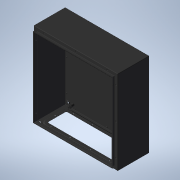
# Autodesk Inventor part: 1050.000(1)_P1
Saved by Autodesk Inventor 2021 (Build 250183000, 183)
## iProperties
Created: 2025-07-29
Part Number: 1050.000(1)_P1
Material: Generic
Catalog Web Link: www.cadenas.de
Description: AE 2.0 Gehaeuse-AE 2.0 Gehaeuse
Vendor: RITTAL
Document SubType Name: Modeling
Designer: psAdmin
Manufacturer: RITTAL
Mass: 833.937 g
Surface Area: 13154.2 cm^2
Volume: 833.937 cm^3
Density: 1 g/cm^3
Appearance: PSOLRGB-176-176-176
Category: PARTsolutions
Company: RITTAL
Title: 1050.000(1)_P1
Author: Cadenas PARTsolutions
Comments: AE 2.0 Gehaeuse
PSOL_IDENT_0: {$CADENAS_DATA/23d-libs/rittal/schaltschranksys/kompakt_schaltschr/parts_ae_2_0/gehaeuse_ae_2_0.prj}
PSOL_IDENT_1: ,190 {VTYP=3D},{NB=1050.000(1)_P1},{LINA=1050.000(1)_P1},{NN=AE 2.0 Gehaeuse},{DATE=25.07.2025 12:41
PSOL_IDENT_2: :23},{GEOMDATE=24.07.2025 05:50:00},{VERSION=},{LINEID=180},{WBVAR=DETAIL},{WBNUMERIC=DETAIL}  {NB=1
PSOL_IDENT_3: 050.000(1)_P1},{LINA=1050.000(1)_P1},{KT=DUMMY},{DETAIL=1},{BEZ1=Neues Kompaktgehäuse},{BEZ2=Stahlbl
PSOL_IDENT_4: ech},{BEZ3=eintürig},{TUER=1},{B=500},{H=500},{T=210},{F=450},{G=475},{B1=500},{BEST=1050.000},{B3=4
PSOL_IDENT_5: 60.000},{B4=383.000},{B5=411.000},{BB5=0.000},{H1=500},{H3=460.000},{H4=85.000},{H5=113.000},{HH5=4.
PSOL_IDENT_6: 000},{T5=93.500},{R1=31.000},{R2=8.000},{T1=210},{F1=450},{G1=475},{VERS3=0},{VERS=4},{CNSECLASS51=2
PSOL_IDENT_7: 7-18-01-02},{CNSECLASS70=27-18-01-01},{CNSECLASS80=27-18-01-01},{CNSETIM40=EC000261},{S=1.25},{W=500
PSOL_IDENT_8: .000},{W1=456.500},{W2=400.000},{HH=500.000},{HH1=456.500},{HH2=450.000},{HH3=375.000},{D=187.000},{
PSOL_IDENT_9: D1=204.300},{VERS1=1},{GEW=15,42},{CNSETIM80=EC000261},{CNSETIM90=EC000261},{CNSECLASS60=27-18-01-01
PSOL_IDENT_10: },{UNSPSC=31-26-15-02}
NB: 1050.000(1)_P1
NN: AE 2.0 Gehaeuse
NT: AE 2.0 Gehaeuse
NBSYN: $BEST.($DETAIL.)_P1
LINA: 1050.000(1)_P1
CATALOG: Rittal
DETAIL: hoch
BEZ1: Neues Kompaktgehäuse
BEZ2: Stahlblech
BEZ3: eintürig
TUER: 1
B: 500
H: 500
T: 210
F: 450
G: 475
B1: 500
BEST: 1050.000
B3: 460
B4: 383
B5: 411
BB5: 0
H1: 500
H3: 460
H4: 85
H5: 113
HH5: 4
T5: 93.5
R1: 31
R2: 8
T1: 210
F1: 450
G1: 475
VERS3: 0
VERS: 4
CNSECLASS70: 27-18-01-01
CNSECLASS80: 27-18-01-01
S: 1.25
W: 500
W1: 456.5
W2: 400
HH: 500
HH1: 456.5
HH2: 450
HH3: 375
D: 187
D1: 204.3
VERS1: 1
GEW: 15,42
CNSETIM80: EC000261
CNSETIM90: EC000261
CNSECLASS60: 27-18-01-01
UNSPSC: 31-26-15-02
SUPPLIER: RITTAL
ARTICLENO: 1050.000(1)_P1
BOMINFO: 1050.000(1)_P1
CREATOR: CADENAS GmbH
Autodesk Inventor part; units mm, degrees
(part 1 of 2)
sketch "Sketch_1" plane through (0, 0, 0) normal (0, 1, 0) x (1, 0, 0)
  line L0 (-250, -82) -> (250, -82)
  line L1 (250, -82) -> (250, 105)
  line L2 (250, 105) -> (-250, 105)
  line L3 (-250, 105) -> (-250, -82)
  arc A0 (-248.75, -79.5) -> (-247.5, -80.75) centre (-247.5, -79.5) ccw
  line L4 (-247.5, -80.75) -> (247.5, -80.75)
  arc A1 (247.5, -80.75) -> (248.75, -79.5) centre (247.5, -79.5) ccw
  line L5 (248.75, -79.5) -> (248.75, 102.5)
  arc A2 (248.75, 102.5) -> (247.5, 103.75) centre (247.5, 102.5) ccw
  line L6 (247.5, 103.75) -> (-247.5, 103.75)
  arc A3 (-247.5, 103.75) -> (-248.75, 102.5) centre (-247.5, 102.5) ccw
  line L7 (-248.75, 102.5) -> (-248.75, -79.5)
  constraints: 16 end point, 8 point on circle, 4 centre point
extrude "Extrusion1" add sketch "Sketch_1" along normal blind 500
sketch "Sketch_2" plane through (0, 0, 82) normal (0, 0, 1) x (1, 0, 0)
  line L0 (-230.75, 19.25) -> (230.75, 19.25)
  line L1 (230.75, 19.25) -> (230.75, 480.75)
  line L2 (230.75, 480.75) -> (-230.75, 480.75)
  line L3 (-230.75, 480.75) -> (-230.75, 19.25)
  constraints: 8 end point
extrude "Extrusion2" cut sketch "Sketch_2" against normal blind 1.25
sketch "Sketch_3" plane through (0, 0, 0) normal (1, 0, 0) x (0, 0, -1)
  line L0 (-82, 490) -> (-80.75, 490)
  line L1 (-80.75, 490) -> (-80.75, 497.5)
  arc A0 (-79.5, 498.75) -> (-80.75, 497.5) centre (-79.5, 497.5) ccw
  line L2 (-79.5, 498.75) -> (102.5, 498.75)
  arc A1 (103.75, 497.5) -> (102.5, 498.75) centre (102.5, 497.5) ccw
  line L3 (103.75, 497.5) -> (103.75, 2.5)
  arc A2 (102.5, 1.25) -> (103.75, 2.5) centre (102.5, 2.5) ccw
  line L4 (102.5, 1.25) -> (-79.5, 1.25)
  arc A3 (-80.75, 2.5) -> (-79.5, 1.25) centre (-79.5, 2.5) ccw
  line L5 (-80.75, 2.5) -> (-80.75, 10)
  line L6 (-80.75, 10) -> (-82, 10)
  line L7 (-82, 10) -> (-82, 0)
  line L8 (-82, 0) -> (105, 0)
  line L9 (105, 0) -> (105, 500)
  line L10 (105, 500) -> (-82, 500)
  line L11 (-82, 500) -> (-82, 490)
  constraints: 24 end point, 8 point on circle, 4 centre point
extrude "Extrusion3" add sketch "Sketch_3" along normal mid plane 500
sketch "Sketch_4" plane through (0, 0, 0) normal (1, 0, 0) x (0, 0, -1)
  line L0 (-83.25, 501.25) -> (-83.25, -1.25)
  line L1 (-83.25, -1.25) -> (106.25, -1.25)
  line L2 (106.25, -1.25) -> (106.25, 501.25)
  line L3 (106.25, 501.25) -> (-83.25, 501.25)
  line L4 (-82, 497.5) -> (-82, 2.5)
  arc A0 (-82, 2.5) -> (-79.5, 0) centre (-79.5, 2.5) ccw
  line L5 (-79.5, 0) -> (102.5, 0)
  arc A1 (102.5, 0) -> (105, 2.5) centre (102.5, 2.5) ccw
  line L6 (105, 2.5) -> (105, 497.5)
  arc A2 (105, 497.5) -> (102.5, 500) centre (102.5, 497.5) ccw
  line L7 (102.5, 500) -> (-79.5, 500)
  arc A3 (-79.5, 500) -> (-82, 497.5) centre (-79.5, 497.5) ccw
  constraints: 16 end point, 8 point on circle, 4 centre point
extrude "Extrusion4" cut sketch "Sketch_4" along normal mid plane 500
sketch "Sketch_5" plane through (0, 0, 0) normal (0, 1, 0) x (1, 0, 0)
  line L0 (-251.25, -83.25) -> (251.25, -83.25)
  line L1 (251.25, -83.25) -> (251.25, 106.25)
  line L2 (251.25, 106.25) -> (-251.25, 106.25)
  line L3 (-251.25, 106.25) -> (-251.25, -83.25)
  arc A0 (-250, -79.5) -> (-247.5, -82) centre (-247.5, -79.5) ccw
  line L4 (-247.5, -82) -> (247.5, -82)
  arc A1 (247.5, -82) -> (250, -79.5) centre (247.5, -79.5) ccw
  line L5 (250, -79.5) -> (250, 102.5)
  arc A2 (250, 102.5) -> (247.5, 105) centre (247.5, 102.5) ccw
  line L6 (247.5, 105) -> (-247.5, 105)
  arc A3 (-247.5, 105) -> (-250, 102.5) centre (-247.5, 102.5) ccw
  line L7 (-250, 102.5) -> (-250, -79.5)
  constraints: 16 end point, 8 point on circle, 4 centre point
extrude "Extrusion5" cut sketch "Sketch_5" along normal blind 500
sketch "Sketch_48" plane through (0, 0, -105) normal (0, 0, 1) x (1, 0, 0)
  line L0 (-246.25, 496.25) -> (-246.25, 3.75)
  line L1 (-246.25, 3.75) -> (246.25, 3.75)
  line L2 (246.25, 3.75) -> (246.25, 496.25)
  line L3 (246.25, 496.25) -> (-246.25, 496.25)
  constraints: 8 end point
extrude "Extrusion6" cut sketch "Sketch_48" along normal blind 1.25
sketch "Sketch_49" plane through (0, 0, -105) normal (0, 0, 1) x (1, 0, 0)
  line L0 (-246.25, 496.25) -> (-246.25, 3.75)
  line L1 (-246.25, 3.75) -> (246.25, 3.75)
  line L2 (246.25, 3.75) -> (246.25, 496.25)
  line L3 (246.25, 496.25) -> (-246.25, 496.25)
  line L4 (218.5, 8.5) -> (241.5, 8.5)
  line L5 (241.5, 8.5) -> (241.5, 31.5)
  line L6 (241.5, 31.5) -> (218.5, 31.5)
  line L7 (218.5, 31.5) -> (218.5, 8.5)
  line L8 (218.5, 468.5) -> (241.5, 468.5)
  line L9 (241.5, 468.5) -> (241.5, 491.5)
  line L10 (241.5, 491.5) -> (218.5, 491.5)
  line L11 (218.5, 491.5) -> (218.5, 468.5)
  line L12 (-241.5, 8.5) -> (-218.5, 8.5)
  line L13 (-218.5, 8.5) -> (-218.5, 31.5)
  line L14 (-218.5, 31.5) -> (-241.5, 31.5)
  line L15 (-241.5, 31.5) -> (-241.5, 8.5)
  line L16 (-241.5, 468.5) -> (-218.5, 468.5)
  line L17 (-218.5, 468.5) -> (-218.5, 491.5)
  line L18 (-218.5, 491.5) -> (-241.5, 491.5)
  line L19 (-241.5, 491.5) -> (-241.5, 468.5)
  constraints: 40 end point
extrude "Extrusion7" add sketch "Sketch_49" along normal blind 1.25
sketch "Sketch_105" plane through (0, 0, -105) normal (0, 0, 1) x (1, 0, 0)
  line L0 (-270, 520) -> (-270, -20)
  line L1 (-270, -20) -> (270, -20)
  line L2 (270, -20) -> (270, 520)
  line L3 (270, 520) -> (-270, 520)
  line L4 (-250, 497.5) -> (-250, 2.5)
  arc A0 (-250, 2.5) -> (-247.5, 0) centre (-247.5, 2.5) ccw
  line L5 (-247.5, 0) -> (247.5, 0)
  arc A1 (247.5, 0) -> (250, 2.5) centre (247.5, 2.5) ccw
  line L6 (250, 2.5) -> (250, 497.5)
  arc A2 (250, 497.5) -> (247.5, 500) centre (247.5, 497.5) ccw
  line L7 (247.5, 500) -> (-247.5, 500)
  arc A3 (-247.5, 500) -> (-250, 497.5) centre (-247.5, 497.5) ccw
  constraints: 16 end point, 8 point on circle, 4 centre point
extrude "Extrusion8" cut sketch "Sketch_105" along normal blind 210
sketch "Sketch_50" plane through (0, 20, 0) normal (0, 1, 0) x (1, 0, 0)
  line L0 (-241.5, 103.75) -> (-240.1443, 103.75)
  line L1 (-240.1443, 103.75) -> (-238.9896, 101.75)
  line L2 (-238.9896, 101.75) -> (-221.0104, 101.75)
  line L3 (-221.0104, 101.75) -> (-219.8557, 103.75)
  line L4 (-219.8557, 103.75) -> (-218.5, 103.75)
  line L5 (-218.5, 103.75) -> (-218.5, 105)
  line L6 (-218.5, 105) -> (-220, 105)
  line L7 (-220, 105) -> (-221.1547, 103)
  line L8 (-221.1547, 103) -> (-238.8453, 103)
  line L9 (-238.8453, 103) -> (-240, 105)
  line L10 (-240, 105) -> (-241.5, 105)
  line L11 (-241.5, 105) -> (-241.5, 103.75)
  constraints: 24 end point
extrude "Extrusion9" add sketch "Sketch_50" along normal mid plane 15.35
sketch "Sketch_51" plane through (0, 20, 0) normal (0, 1, 0) x (1, 0, 0)
  line L0 (218.5, 103.75) -> (219.8557, 103.75)
  line L1 (219.8557, 103.75) -> (221.0104, 101.75)
  line L2 (221.0104, 101.75) -> (238.9896, 101.75)
  line L3 (238.9896, 101.75) -> (240.1443, 103.75)
  line L4 (240.1443, 103.75) -> (241.5, 103.75)
  line L5 (241.5, 103.75) -> (241.5, 105)
  line L6 (241.5, 105) -> (240, 105)
  line L7 (240, 105) -> (238.8453, 103)
  line L8 (238.8453, 103) -> (221.1547, 103)
  line L9 (221.1547, 103) -> (220, 105)
  line L10 (220, 105) -> (218.5, 105)
  line L11 (218.5, 105) -> (218.5, 103.75)
  constraints: 24 end point
extrude "Extrusion10" add sketch "Sketch_51" along normal mid plane 15.35
sketch "Sketch_52" plane through (0, 27.675, 0) normal (0, 1, 0) x (1, 0, 0)
  line L0 (-222.325, 101.75) -> (-222.325, 103)
  line L1 (-222.325, 103) -> (-221.1547, 103)
  line L2 (-221.1547, 103) -> (-220, 105)
  line L3 (-220, 105) -> (-215.5, 105)
  line L4 (-215.5, 105) -> (-215.5, 103.75)
  line L5 (-215.5, 103.75) -> (-219.8557, 103.75)
  line L6 (-219.8557, 103.75) -> (-221.0104, 101.75)
  line L7 (-221.0104, 101.75) -> (-222.325, 101.75)
  line L8 (-222.325, 101.75) -> (-222.325, 103)
  constraints: 18 end point
revolve "Revolution1" add sketch "Sketch_52" angle 90 about axis through (-222.325, 27.675, -101.75) along (0, 0, 1)
sketch "Sketch_53" plane through (0, 27.675, 0) normal (0, 1, 0) x (1, 0, 0)
  line L0 (-237.675, 103) -> (-237.675, 101.75)
  line L1 (-237.675, 101.75) -> (-238.9896, 101.75)
  line L2 (-238.9896, 101.75) -> (-240.1443, 103.75)
  line L3 (-240.1443, 103.75) -> (-244.5, 103.75)
  line L4 (-244.5, 103.75) -> (-244.5, 105)
  line L5 (-244.5, 105) -> (-240, 105)
  line L6 (-240, 105) -> (-238.8453, 103)
  line L7 (-238.8453, 103) -> (-237.675, 103)
  line L8 (-237.675, 103) -> (-237.675, 101.75)
  constraints: 18 end point
revolve "Revolution2" add sketch "Sketch_53" angle 90 about axis through (-237.675, 27.675, -103) along (0, 0, -1)
sketch "Sketch_54" plane through (0, 27.675, 0) normal (0, 1, 0) x (1, 0, 0)
  line L0 (237.675, 101.75) -> (237.675, 103)
  line L1 (237.675, 103) -> (238.8453, 103)
  line L2 (238.8453, 103) -> (240, 105)
  line L3 (240, 105) -> (244.5, 105)
  line L4 (244.5, 105) -> (244.5, 103.75)
  line L5 (244.5, 103.75) -> (240.1443, 103.75)
  line L6 (240.1443, 103.75) -> (238.9896, 101.75)
  line L7 (238.9896, 101.75) -> (237.675, 101.75)
  line L8 (237.675, 101.75) -> (237.675, 103)
  constraints: 18 end point
revolve "Revolution3" add sketch "Sketch_54" angle 90 about axis through (237.675, 27.675, -101.75) along (0, 0, 1)
sketch "Sketch_55" plane through (0, 27.675, 0) normal (0, 1, 0) x (1, 0, 0)
  line L0 (222.325, 103) -> (222.325, 101.75)
  line L1 (222.325, 101.75) -> (221.0104, 101.75)
  line L2 (221.0104, 101.75) -> (219.8557, 103.75)
  line L3 (219.8557, 103.75) -> (215.5, 103.75)
  line L4 (215.5, 103.75) -> (215.5, 105)
  line L5 (215.5, 105) -> (220, 105)
  line L6 (220, 105) -> (221.1547, 103)
  line L7 (221.1547, 103) -> (222.325, 103)
  line L8 (222.325, 103) -> (222.325, 101.75)
  constraints: 18 end point
revolve "Revolution4" add sketch "Sketch_55" angle 90 about axis through (222.325, 27.675, -103) along (0, 0, -1)
sketch "Sketch_56" plane through (0, 12.325, 0) normal (0, 1, 0) x (1, 0, 0)
  line L0 (-222.325, 101.75) -> (-222.325, 103)
  line L1 (-222.325, 103) -> (-221.1547, 103)
  line L2 (-221.1547, 103) -> (-220, 105)
  line L3 (-220, 105) -> (-215.5, 105)
  line L4 (-215.5, 105) -> (-215.5, 103.75)
  line L5 (-215.5, 103.75) -> (-219.8557, 103.75)
  line L6 (-219.8557, 103.75) -> (-221.0104, 101.75)
  line L7 (-221.0104, 101.75) -> (-222.325, 101.75)
  line L8 (-222.325, 101.75) -> (-222.325, 103)
  constraints: 18 end point
revolve "Revolution5" add sketch "Sketch_56" angle 90 about axis through (-222.325, 12.325, -101.75) along (0, 0, -1)
sketch "Sketch_57" plane through (0, 12.325, 0) normal (0, 1, 0) x (1, 0, 0)
  line L0 (-237.675, 103) -> (-237.675, 101.75)
  line L1 (-237.675, 101.75) -> (-238.9896, 101.75)
  line L2 (-238.9896, 101.75) -> (-240.1443, 103.75)
  line L3 (-240.1443, 103.75) -> (-244.5, 103.75)
  line L4 (-244.5, 103.75) -> (-244.5, 105)
  line L5 (-244.5, 105) -> (-240, 105)
  line L6 (-240, 105) -> (-238.8453, 103)
  line L7 (-238.8453, 103) -> (-237.675, 103)
  line L8 (-237.675, 103) -> (-237.675, 101.75)
  constraints: 18 end point
revolve "Revolution6" add sketch "Sketch_57" angle 90 about axis through (-237.675, 12.325, -103) along (0, 0, 1)
sketch "Sketch_58" plane through (0, 12.325, 0) normal (0, 1, 0) x (1, 0, 0)
  line L0 (237.675, 101.75) -> (237.675, 103)
  line L1 (237.675, 103) -> (238.8453, 103)
  line L2 (238.8453, 103) -> (240, 105)
  line L3 (240, 105) -> (244.5, 105)
  line L4 (244.5, 105) -> (244.5, 103.75)
  line L5 (244.5, 103.75) -> (240.1443, 103.75)
  line L6 (240.1443, 103.75) -> (238.9896, 101.75)
  line L7 (238.9896, 101.75) -> (237.675, 101.75)
  line L8 (237.675, 101.75) -> (237.675, 103)
  constraints: 18 end point
revolve "Revolution7" add sketch "Sketch_58" angle 90 about axis through (237.675, 12.325, -101.75) along (0, 0, -1)
sketch "Sketch_59" plane through (0, 12.325, 0) normal (0, 1, 0) x (1, 0, 0)
  line L0 (222.325, 103) -> (222.325, 101.75)
  line L1 (222.325, 101.75) -> (221.0104, 101.75)
  line L2 (221.0104, 101.75) -> (219.8557, 103.75)
  line L3 (219.8557, 103.75) -> (215.5, 103.75)
  line L4 (215.5, 103.75) -> (215.5, 105)
  line L5 (215.5, 105) -> (220, 105)
  line L6 (220, 105) -> (221.1547, 103)
  line L7 (221.1547, 103) -> (222.325, 103)
  line L8 (222.325, 103) -> (222.325, 101.75)
  constraints: 18 end point
revolve "Revolution8" add sketch "Sketch_59" angle 90 about axis through (222.325, 12.325, -103) along (0, 0, 1)
sketch "Sketch_60" plane through (0, 480, 0) normal (0, 1, 0) x (1, 0, 0)
  line L0 (-241.5, 103.75) -> (-240.1443, 103.75)
  line L1 (-240.1443, 103.75) -> (-238.9896, 101.75)
  line L2 (-238.9896, 101.75) -> (-221.0104, 101.75)
  line L3 (-221.0104, 101.75) -> (-219.8557, 103.75)
  line L4 (-219.8557, 103.75) -> (-218.5, 103.75)
  line L5 (-218.5, 103.75) -> (-218.5, 105)
  line L6 (-218.5, 105) -> (-220, 105)
  line L7 (-220, 105) -> (-221.1547, 103)
  line L8 (-221.1547, 103) -> (-238.8453, 103)
  line L9 (-238.8453, 103) -> (-240, 105)
  line L10 (-240, 105) -> (-241.5, 105)
  line L11 (-241.5, 105) -> (-241.5, 103.75)
  constraints: 24 end point
extrude "Extrusion11" add sketch "Sketch_60" along normal mid plane 15.35
sketch "Sketch_61" plane through (0, 480, 0) normal (0, 1, 0) x (1, 0, 0)
  line L0 (218.5, 103.75) -> (219.8557, 103.75)
  line L1 (219.8557, 103.75) -> (221.0104, 101.75)
  line L2 (221.0104, 101.75) -> (238.9896, 101.75)
  line L3 (238.9896, 101.75) -> (240.1443, 103.75)
  line L4 (240.1443, 103.75) -> (241.5, 103.75)
  line L5 (241.5, 103.75) -> (241.5, 105)
  line L6 (241.5, 105) -> (240, 105)
  line L7 (240, 105) -> (238.8453, 103)
  line L8 (238.8453, 103) -> (221.1547, 103)
  line L9 (221.1547, 103) -> (220, 105)
  line L10 (220, 105) -> (218.5, 105)
  line L11 (218.5, 105) -> (218.5, 103.75)
  constraints: 24 end point
extrude "Extrusion12" add sketch "Sketch_61" along normal mid plane 15.35
sketch "Sketch_62" plane through (0, 487.675, 0) normal (0, 1, 0) x (1, 0, 0)
  line L0 (-222.325, 101.75) -> (-222.325, 103)
  line L1 (-222.325, 103) -> (-221.1547, 103)
  line L2 (-221.1547, 103) -> (-220, 105)
  line L3 (-220, 105) -> (-215.5, 105)
  line L4 (-215.5, 105) -> (-215.5, 103.75)
  line L5 (-215.5, 103.75) -> (-219.8557, 103.75)
  line L6 (-219.8557, 103.75) -> (-221.0104, 101.75)
  line L7 (-221.0104, 101.75) -> (-222.325, 101.75)
  line L8 (-222.325, 101.75) -> (-222.325, 103)
  constraints: 18 end point
revolve "Revolution9" add sketch "Sketch_62" angle 90 about axis through (-222.325, 487.675, -101.75) along (0, 0, 1)
sketch "Sketch_63" plane through (0, 487.675, 0) normal (0, 1, 0) x (1, 0, 0)
  line L0 (-237.675, 103) -> (-237.675, 101.75)
  line L1 (-237.675, 101.75) -> (-238.9896, 101.75)
  line L2 (-238.9896, 101.75) -> (-240.1443, 103.75)
  line L3 (-240.1443, 103.75) -> (-244.5, 103.75)
  line L4 (-244.5, 103.75) -> (-244.5, 105)
  line L5 (-244.5, 105) -> (-240, 105)
  line L6 (-240, 105) -> (-238.8453, 103)
  line L7 (-238.8453, 103) -> (-237.675, 103)
  line L8 (-237.675, 103) -> (-237.675, 101.75)
  constraints: 18 end point
revolve "Revolution10" add sketch "Sketch_63" angle 90 about axis through (-237.675, 487.675, -103) along (0, 0, -1)
sketch "Sketch_64" plane through (0, 487.675, 0) normal (0, 1, 0) x (1, 0, 0)
  line L0 (237.675, 101.75) -> (237.675, 103)
  line L1 (237.675, 103) -> (238.8453, 103)
  line L2 (238.8453, 103) -> (240, 105)
  line L3 (240, 105) -> (244.5, 105)
  line L4 (244.5, 105) -> (244.5, 103.75)
  line L5 (244.5, 103.75) -> (240.1443, 103.75)
  line L6 (240.1443, 103.75) -> (238.9896, 101.75)
  line L7 (238.9896, 101.75) -> (237.675, 101.75)
  line L8 (237.675, 101.75) -> (237.675, 103)
  constraints: 18 end point
revolve "Revolution11" add sketch "Sketch_64" angle 90 about axis through (237.675, 487.675, -101.75) along (0, 0, 1)
sketch "Sketch_65" plane through (0, 487.675, 0) normal (0, 1, 0) x (1, 0, 0)
  line L0 (222.325, 103) -> (222.325, 101.75)
  line L1 (222.325, 101.75) -> (221.0104, 101.75)
  line L2 (221.0104, 101.75) -> (219.8557, 103.75)
  line L3 (219.8557, 103.75) -> (215.5, 103.75)
  line L4 (215.5, 103.75) -> (215.5, 105)
  line L5 (215.5, 105) -> (220, 105)
  line L6 (220, 105) -> (221.1547, 103)
  line L7 (221.1547, 103) -> (222.325, 103)
  line L8 (222.325, 103) -> (222.325, 101.75)
  constraints: 18 end point
revolve "Revolution12" add sketch "Sketch_65" angle 90 about axis through (222.325, 487.675, -103) along (0, 0, -1)
sketch "Sketch_66" plane through (0, 472.325, 0) normal (0, 1, 0) x (1, 0, 0)
  line L0 (-222.325, 101.75) -> (-222.325, 103)
  line L1 (-222.325, 103) -> (-221.1547, 103)
  line L2 (-221.1547, 103) -> (-220, 105)
  line L3 (-220, 105) -> (-215.5, 105)
  line L4 (-215.5, 105) -> (-215.5, 103.75)
  line L5 (-215.5, 103.75) -> (-219.8557, 103.75)
  line L6 (-219.8557, 103.75) -> (-221.0104, 101.75)
  line L7 (-221.0104, 101.75) -> (-222.325, 101.75)
  line L8 (-222.325, 101.75) -> (-222.325, 103)
  constraints: 18 end point
revolve "Revolution13" add sketch "Sketch_66" angle 90 about axis through (-222.325, 472.325, -101.75) along (0, 0, -1)
sketch "Sketch_67" plane through (0, 472.325, 0) normal (0, 1, 0) x (1, 0, 0)
  line L0 (-237.675, 103) -> (-237.675, 101.75)
  line L1 (-237.675, 101.75) -> (-238.9896, 101.75)
  line L2 (-238.9896, 101.75) -> (-240.1443, 103.75)
  line L3 (-240.1443, 103.75) -> (-244.5, 103.75)
  line L4 (-244.5, 103.75) -> (-244.5, 105)
  line L5 (-244.5, 105) -> (-240, 105)
  line L6 (-240, 105) -> (-238.8453, 103)
  line L7 (-238.8453, 103) -> (-237.675, 103)
  line L8 (-237.675, 103) -> (-237.675, 101.75)
  constraints: 18 end point
revolve "Revolution14" add sketch "Sketch_67" angle 90 about axis through (-237.675, 472.325, -103) along (0, 0, 1)
sketch "Sketch_68" plane through (0, 472.325, 0) normal (0, 1, 0) x (1, 0, 0)
  line L0 (237.675, 101.75) -> (237.675, 103)
  line L1 (237.675, 103) -> (238.8453, 103)
  line L2 (238.8453, 103) -> (240, 105)
  line L3 (240, 105) -> (244.5, 105)
  line L4 (244.5, 105) -> (244.5, 103.75)
  line L5 (244.5, 103.75) -> (240.1443, 103.75)
  line L6 (240.1443, 103.75) -> (238.9896, 101.75)
  line L7 (238.9896, 101.75) -> (237.675, 101.75)
  line L8 (237.675, 101.75) -> (237.675, 103)
  constraints: 18 end point
revolve "Revolution15" add sketch "Sketch_68" angle 90 about axis through (237.675, 472.325, -101.75) along (0, 0, -1)
sketch "Sketch_69" plane through (0, 472.325, 0) normal (0, 1, 0) x (1, 0, 0)
  line L0 (222.325, 103) -> (222.325, 101.75)
  line L1 (222.325, 101.75) -> (221.0104, 101.75)
  line L2 (221.0104, 101.75) -> (219.8557, 103.75)
  line L3 (219.8557, 103.75) -> (215.5, 103.75)
  line L4 (215.5, 103.75) -> (215.5, 105)
  line L5 (215.5, 105) -> (220, 105)
  line L6 (220, 105) -> (221.1547, 103)
  line L7 (221.1547, 103) -> (222.325, 103)
  line L8 (222.325, 103) -> (222.325, 101.75)
  constraints: 18 end point
revolve "Revolution16" add sketch "Sketch_69" angle 90 about axis through (222.325, 472.325, -103) along (0, 0, 1)
sketch "Sketch_70" plane through (-230, 0, 0) normal (1, 0, 0) x (0, 0, -1)
  line L0 (101.75, 11.0104) -> (103.75, 9.8557)
  line L1 (103.75, 9.8557) -> (103.75, 8.5)
  line L2 (103.75, 8.5) -> (105, 8.5)
  line L3 (105, 8.5) -> (105, 10)
  line L4 (105, 10) -> (103, 11.1547)
  line L5 (103, 11.1547) -> (103, 28.8453)
  line L6 (103, 28.8453) -> (105, 30)
  line L7 (105, 30) -> (105, 31.5)
  line L8 (105, 31.5) -> (103.75, 31.5)
  line L9 (103.75, 31.5) -> (103.75, 30.1443)
  line L10 (103.75, 30.1443) -> (101.75, 28.9896)
  line L11 (101.75, 28.9896) -> (101.75, 11.0104)
  constraints: 24 end point
extrude "Extrusion13" add sketch "Sketch_70" along normal mid plane 15.35
sketch "Sketch_71" plane through (-230, 0, 0) normal (1, 0, 0) x (0, 0, -1)
  line L0 (101.75, 471.0104) -> (103.75, 469.8557)
  line L1 (103.75, 469.8557) -> (103.75, 468.5)
  line L2 (103.75, 468.5) -> (105, 468.5)
  line L3 (105, 468.5) -> (105, 470)
  line L4 (105, 470) -> (103, 471.1547)
  line L5 (103, 471.1547) -> (103, 488.8453)
  line L6 (103, 488.8453) -> (105, 490)
  line L7 (105, 490) -> (105, 491.5)
  line L8 (105, 491.5) -> (103.75, 491.5)
  line L9 (103.75, 491.5) -> (103.75, 490.1443)
  line L10 (103.75, 490.1443) -> (101.75, 488.9896)
  line L11 (101.75, 488.9896) -> (101.75, 471.0104)
  constraints: 24 end point
extrude "Extrusion14" add sketch "Sketch_71" along normal mid plane 15.35
sketch "Sketch_74" plane through (-230, 0, 0) normal (1, 0, 0) x (0, 0, -1)
  line L0 (104.5, 20) -> (101.75, 20)
  line L1 (101.75, 20) -> (101.75, 26.25)
  line L2 (101.75, 26.25) -> (103, 26.25)
  line L3 (103, 26.25) -> (103, 25.6)
  line L4 (103, 25.6) -> (104.5, 25.6)
  line L5 (104.5, 25.6) -> (104.5, 20)
  line L6 (104.5, 20) -> (101.75, 20)
  constraints: 14 end point
revolve "Revolution17" add sketch "Sketch_74" angle 360 about axis through (-230, 20, -104.5) along (0, 0, 1)
sketch "Sketch_75" plane through (-230, 0, 0) normal (1, 0, 0) x (0, 0, -1)
  line L0 (105, 20) -> (101.25, 20)
  line L1 (101.25, 20) -> (101.25, 25.625)
  line L2 (101.25, 25.625) -> (101.75, 25.625)
  arc A0 (101.75, 25.625) -> (102.75, 24.625) centre (102.75, 25.625) ccw
  line L3 (102.75, 24.625) -> (104.3, 24.625)
  arc A1 (104.3, 24.625) -> (104.5, 24.825) centre (104.3, 24.825) ccw
  line L4 (104.5, 24.825) -> (104.5, 25.625)
  line L5 (104.5, 25.625) -> (105, 25.625)
  line L6 (105, 25.625) -> (105, 20)
  line L7 (105, 20) -> (101.25, 20)
  constraints: 16 end point, 4 point on circle, 2 centre point
revolve "Revolution18" cut sketch "Sketch_75" angle 360 about axis through (-230, 20, -105) along (0, 0, 1)
sketch "Sketch_76" plane through (-230, 0, 0) normal (1, 0, 0) x (0, 0, -1)
  line L0 (104.5, 480) -> (101.75, 480)
  line L1 (101.75, 480) -> (101.75, 486.25)
  line L2 (101.75, 486.25) -> (103, 486.25)
  line L3 (103, 486.25) -> (103, 485.6)
  line L4 (103, 485.6) -> (104.5, 485.6)
  line L5 (104.5, 485.6) -> (104.5, 480)
  line L6 (104.5, 480) -> (101.75, 480)
  constraints: 14 end point
revolve "Revolution19" add sketch "Sketch_76" angle 360 about axis through (-230, 480, -104.5) along (0, 0, 1)
sketch "Sketch_77" plane through (-230, 0, 0) normal (1, 0, 0) x (0, 0, -1)
  line L0 (105, 480) -> (101.25, 480)
  line L1 (101.25, 480) -> (101.25, 485.625)
  line L2 (101.25, 485.625) -> (101.75, 485.625)
  arc A0 (101.75, 485.625) -> (102.75, 484.625) centre (102.75, 485.625) ccw
  line L3 (102.75, 484.625) -> (104.3, 484.625)
  arc A1 (104.3, 484.625) -> (104.5, 484.825) centre (104.3, 484.825) ccw
  line L4 (104.5, 484.825) -> (104.5, 485.625)
  line L5 (104.5, 485.625) -> (105, 485.625)
  line L6 (105, 485.625) -> (105, 480)
  line L7 (105, 480) -> (101.25, 480)
  constraints: 16 end point, 4 point on circle, 2 centre point
revolve "Revolution20" cut sketch "Sketch_77" angle 360 about axis through (-230, 480, -105) along (0, 0, 1)
sketch "Sketch_72" plane through (230, 0, 0) normal (1, 0, 0) x (0, 0, -1)
  line L0 (101.75, 11.0104) -> (103.75, 9.8557)
  line L1 (103.75, 9.8557) -> (103.75, 8.5)
  line L2 (103.75, 8.5) -> (105, 8.5)
  line L3 (105, 8.5) -> (105, 10)
  line L4 (105, 10) -> (103, 11.1547)
  line L5 (103, 11.1547) -> (103, 28.8453)
  line L6 (103, 28.8453) -> (105, 30)
  line L7 (105, 30) -> (105, 31.5)
  line L8 (105, 31.5) -> (103.75, 31.5)
  line L9 (103.75, 31.5) -> (103.75, 30.1443)
  line L10 (103.75, 30.1443) -> (101.75, 28.9896)
  line L11 (101.75, 28.9896) -> (101.75, 11.0104)
  constraints: 24 end point
extrude "Extrusion15" add sketch "Sketch_72" along normal mid plane 15.35
sketch "Sketch_73" plane through (230, 0, 0) normal (1, 0, 0) x (0, 0, -1)
  line L0 (101.75, 471.0104) -> (103.75, 469.8557)
  line L1 (103.75, 469.8557) -> (103.75, 468.5)
  line L2 (103.75, 468.5) -> (105, 468.5)
  line L3 (105, 468.5) -> (105, 470)
  line L4 (105, 470) -> (103, 471.1547)
  line L5 (103, 471.1547) -> (103, 488.8453)
  line L6 (103, 488.8453) -> (105, 490)
  line L7 (105, 490) -> (105, 491.5)
  line L8 (105, 491.5) -> (103.75, 491.5)
  line L9 (103.75, 491.5) -> (103.75, 490.1443)
  line L10 (103.75, 490.1443) -> (101.75, 488.9896)
  line L11 (101.75, 488.9896) -> (101.75, 471.0104)
  constraints: 24 end point
extrude "Extrusion16" add sketch "Sketch_73" along normal mid plane 15.35
sketch "Sketch_78" plane through (230, 0, 0) normal (1, 0, 0) x (0, 0, -1)
  line L0 (104.5, 20) -> (101.75, 20)
  line L1 (101.75, 20) -> (101.75, 26.25)
  line L2 (101.75, 26.25) -> (103, 26.25)
  line L3 (103, 26.25) -> (103, 25.6)
  line L4 (103, 25.6) -> (104.5, 25.6)
  line L5 (104.5, 25.6) -> (104.5, 20)
  line L6 (104.5, 20) -> (101.75, 20)
  constraints: 14 end point
revolve "Revolution21" add sketch "Sketch_78" angle 360 about axis through (230, 20, -104.5) along (0, 0, 1)
sketch "Sketch_79" plane through (230, 0, 0) normal (1, 0, 0) x (0, 0, -1)
  line L0 (105, 20) -> (101.25, 20)
  line L1 (101.25, 20) -> (101.25, 25.625)
  line L2 (101.25, 25.625) -> (101.75, 25.625)
  arc A0 (101.75, 25.625) -> (102.75, 24.625) centre (102.75, 25.625) ccw
  line L3 (102.75, 24.625) -> (104.3, 24.625)
  arc A1 (104.3, 24.625) -> (104.5, 24.825) centre (104.3, 24.825) ccw
  line L4 (104.5, 24.825) -> (104.5, 25.625)
  line L5 (104.5, 25.625) -> (105, 25.625)
  line L6 (105, 25.625) -> (105, 20)
  line L7 (105, 20) -> (101.25, 20)
  constraints: 16 end point, 4 point on circle, 2 centre point
revolve "Revolution22" cut sketch "Sketch_79" angle 360 about axis through (230, 20, -105) along (0, 0, 1)
sketch "Sketch_80" plane through (230, 0, 0) normal (1, 0, 0) x (0, 0, -1)
  line L0 (104.5, 480) -> (101.75, 480)
  line L1 (101.75, 480) -> (101.75, 486.25)
  line L2 (101.75, 486.25) -> (103, 486.25)
  line L3 (103, 486.25) -> (103, 485.6)
  line L4 (103, 485.6) -> (104.5, 485.6)
  line L5 (104.5, 485.6) -> (104.5, 480)
  line L6 (104.5, 480) -> (101.75, 480)
  constraints: 14 end point
revolve "Revolution23" add sketch "Sketch_80" angle 360 about axis through (230, 480, -104.5) along (0, 0, 1)
sketch "Sketch_81" plane through (230, 0, 0) normal (1, 0, 0) x (0, 0, -1)
  line L0 (105, 480) -> (101.25, 480)
  line L1 (101.25, 480) -> (101.25, 485.625)
  line L2 (101.25, 485.625) -> (101.75, 485.625)
  arc A0 (101.75, 485.625) -> (102.75, 484.625) centre (102.75, 485.625) ccw
  line L3 (102.75, 484.625) -> (104.3, 484.625)
  arc A1 (104.3, 484.625) -> (104.5, 484.825) centre (104.3, 484.825) ccw
  line L4 (104.5, 484.825) -> (104.5, 485.625)
  line L5 (104.5, 485.625) -> (105, 485.625)
  line L6 (105, 485.625) -> (105, 480)
  line L7 (105, 480) -> (101.25, 480)
  constraints: 16 end point, 4 point on circle, 2 centre point
revolve "Revolution24" cut sketch "Sketch_81" angle 360 about axis through (230, 480, -105) along (0, 0, 1)
sketch "Sketch_6" plane through (0, 0, 0) normal (1, 0, 0) x (0, 0, -1)
  line L0 (-99.3, 485.9911) -> (-98.8224, 480.5321)
  arc A0 (-98.8224, 480.5321) -> (-96.3319, 478.25) centre (-96.3319, 480.75) ccw
  line L1 (-96.3319, 478.25) -> (-83.25, 478.25)
  arc A1 (-83.25, 478.25) -> (-80.75, 480.75) centre (-83.25, 480.75) ccw
  line L2 (-80.75, 480.75) -> (-80.75, 486.1)
  line L3 (-80.75, 486.1) -> (-98.0548, 486.1)
  line L4 (-98.0548, 486.1) -> (-99.3, 485.9911)
  constraints: 10 end point, 4 point on circle, 2 centre point
extrude "Extrusion17" add sketch "Sketch_6" along normal mid plane 474.2
sketch "Sketch_7" plane through (0, 0, 0) normal (1, 0, 0) x (0, 0, -1)
  line L0 (-99.3, 14.0089) -> (-98.0548, 13.9)
  line L1 (-98.0548, 13.9) -> (-80.75, 13.9)
  line L2 (-80.75, 13.9) -> (-80.75, 19.25)
  arc A0 (-80.75, 19.25) -> (-83.25, 21.75) centre (-83.25, 19.25) ccw
  line L3 (-83.25, 21.75) -> (-96.3319, 21.75)
  arc A1 (-96.3319, 21.75) -> (-98.8224, 19.4679) centre (-96.3319, 19.25) ccw
  line L4 (-98.8224, 19.4679) -> (-99.3, 14.0089)
  constraints: 10 end point, 4 point on circle, 2 centre point
extrude "Extrusion18" add sketch "Sketch_7" along normal mid plane 474.2
sketch "Sketch_8" plane through (0, 250, 0) normal (0, 1, 0) x (1, 0, 0)
  line L0 (228.25, -83.25) -> (228.25, -96.3319)
  arc A0 (228.25, -96.3319) -> (230.5321, -98.8224) centre (230.75, -96.3319) ccw
  line L1 (230.5321, -98.8224) -> (235.9911, -99.3)
  line L2 (235.9911, -99.3) -> (236.1, -98.0548)
  line L3 (236.1, -98.0548) -> (236.1, -80.75)
  line L4 (236.1, -80.75) -> (230.75, -80.75)
  arc A1 (230.75, -80.75) -> (228.25, -83.25) centre (230.75, -83.25) ccw
  constraints: 10 end point, 4 point on circle, 2 centre point
extrude "Extrusion19" add sketch "Sketch_8" along normal mid plane 474.2
sketch "Sketch_9" plane through (0, 250, 0) normal (0, 1, 0) x (1, 0, 0)
  line L0 (-236.1, -98.0548) -> (-235.9911, -99.3)
  line L1 (-235.9911, -99.3) -> (-230.5321, -98.8224)
  arc A0 (-230.5321, -98.8224) -> (-228.25, -96.3319) centre (-230.75, -96.3319) ccw
  line L2 (-228.25, -96.3319) -> (-228.25, -83.25)
  arc A1 (-228.25, -83.25) -> (-230.75, -80.75) centre (-230.75, -83.25) ccw
  line L3 (-230.75, -80.75) -> (-236.1, -80.75)
  line L4 (-236.1, -80.75) -> (-236.1, -98.0548)
  constraints: 10 end point, 4 point on circle, 2 centre point
extrude "Extrusion20" add sketch "Sketch_9" along normal mid plane 474.2
sketch "Sketch_12" plane through (0, 250, 0) normal (0, 1, 0) x (1, 0, 0)
  line L0 (-237.35, -82) -> (-237.35, -101.8)
  line L1 (-237.35, -101.8) -> (237.35, -101.8)
  line L2 (237.35, -101.8) -> (237.35, -82)
  line L3 (237.35, -82) -> (230.75, -82)
  arc A0 (230.75, -82) -> (229.5, -83.25) centre (230.75, -83.25) ccw
  line L4 (229.5, -83.25) -> (229.5, -96.3319)
  arc A1 (229.5, -96.3319) -> (230.6411, -97.5772) centre (230.75, -96.3319) ccw
  line L5 (230.6411, -97.5772) -> (236.1, -98.0548)
  line L6 (236.1, -98.0548) -> (235.9911, -99.3)
  line L7 (235.9911, -99.3) -> (-235.9911, -99.3)
  line L8 (-235.9911, -99.3) -> (-236.1, -98.0548)
  line L9 (-236.1, -98.0548) -> (-230.6411, -97.5772)
  arc A2 (-230.6411, -97.5772) -> (-229.5, -96.3319) centre (-230.75, -96.3319) ccw
  line L10 (-229.5, -96.3319) -> (-229.5, -83.25)
  arc A3 (-229.5, -83.25) -> (-230.75, -82) centre (-230.75, -83.25) ccw
  line L11 (-230.75, -82) -> (-237.35, -82)
  constraints: 24 end point, 8 point on circle, 4 centre point
extrude "Extrusion21" cut sketch "Sketch_12" along normal mid plane 472.2
sketch "Sketch_11" plane through (0, 0, 0) normal (1, 0, 0) x (0, 0, -1)
  line L0 (-101.8, 11.4) -> (-82, 11.4)
  line L1 (-82, 11.4) -> (-82, 19.25)
  arc A0 (-82, 19.25) -> (-83.25, 20.5) centre (-83.25, 19.25) ccw
  line L2 (-83.25, 20.5) -> (-96.3319, 20.5)
  arc A1 (-96.3319, 20.5) -> (-97.5772, 19.3589) centre (-96.3319, 19.25) ccw
  line L3 (-97.5772, 19.3589) -> (-98.0548, 13.9)
  line L4 (-98.0548, 13.9) -> (-99.3, 14.0089)
  line L5 (-99.3, 14.0089) -> (-99.3, 485.9911)
  line L6 (-99.3, 485.9911) -> (-98.0548, 486.1)
  line L7 (-98.0548, 486.1) -> (-97.5772, 480.6411)
  arc A2 (-97.5772, 480.6411) -> (-96.3319, 479.5) centre (-96.3319, 480.75) ccw
  line L8 (-96.3319, 479.5) -> (-83.25, 479.5)
  arc A3 (-83.25, 479.5) -> (-82, 480.75) centre (-83.25, 480.75) ccw
  line L9 (-82, 480.75) -> (-82, 488.6)
  line L10 (-82, 488.6) -> (-101.8, 488.6)
  line L11 (-101.8, 488.6) -> (-101.8, 11.4)
  constraints: 24 end point, 8 point on circle, 4 centre point
extrude "Extrusion22" cut sketch "Sketch_11" along normal mid plane 472.2
sketch "Sketch_13" plane through (0, 475, 0) normal (0, 1, 0) x (1, 0, 0)
  line L0 (-200, 72.75) -> (-200, 103.75)
  line L1 (-200, 103.75) -> (-193.5, 103.75)
  line L2 (-193.5, 103.75) -> (-193.5, 102.75)
  line L3 (-193.5, 102.75) -> (-192.45, 102.75)
  line L4 (-192.45, 102.75) -> (-192.25, 102.55)
  line L5 (-192.25, 102.55) -> (-192.25, 93.55)
  arc A0 (-192.55, 93.25) -> (-192.25, 93.55) centre (-192.55, 93.55) ccw
  line L6 (-192.55, 93.25) -> (-192.25, 93.25)
  line L7 (-192.25, 93.25) -> (-192.25, 87.75)
  line L8 (-192.25, 87.75) -> (-196, 87.75)
  line L9 (-196, 87.75) -> (-196, 85)
  line L10 (-196, 85) -> (-191, 85)
  arc A1 (-190.8875, 82.5051) -> (-191, 85) centre (-191, 83.75) ccw
  line L11 (-190.8875, 82.5051) -> (-192.2, 82.3864)
  line L12 (-192.2, 82.3864) -> (-192.2, 77.3483)
  line L13 (-192.2, 77.3483) -> (-193.5, 77)
  line L14 (-193.5, 77) -> (-196, 77)
  line L15 (-196, 77) -> (-196, 73.517)
  line L16 (-196, 73.517) -> (-196.767, 72.75)
  line L17 (-196.767, 72.75) -> (-200, 72.75)
  line L18 (-200, 72.75) -> (-200, 103.75)
  constraints: 38 end point, 4 point on circle, 2 centre point
revolve "Revolution25" add sketch "Sketch_13" angle 360 about axis through (-200, 475, -72.75) along (0, 0, 1)
thread "Thread1" size "M8x1.25" class "6g" standard "ISO Metric profile" length 1.4216
sketch "Sketch_14" plane through (0, 475, 0) normal (0, 1, 0) x (1, 0, 0)
  line L0 (200, 72.75) -> (200, 103.75)
  line L1 (200, 103.75) -> (206.5, 103.75)
  line L2 (206.5, 103.75) -> (206.5, 102.75)
  line L3 (206.5, 102.75) -> (207.55, 102.75)
  line L4 (207.55, 102.75) -> (207.75, 102.55)
  line L5 (207.75, 102.55) -> (207.75, 93.55)
  arc A0 (207.45, 93.25) -> (207.75, 93.55) centre (207.45, 93.55) ccw
  line L6 (207.45, 93.25) -> (207.75, 93.25)
  line L7 (207.75, 93.25) -> (207.75, 87.75)
  line L8 (207.75, 87.75) -> (204, 87.75)
  line L9 (204, 87.75) -> (204, 85)
  line L10 (204, 85) -> (209, 85)
  arc A1 (209.1125, 82.5051) -> (209, 85) centre (209, 83.75) ccw
  line L11 (209.1125, 82.5051) -> (207.8, 82.3864)
  line L12 (207.8, 82.3864) -> (207.8, 77.3483)
  line L13 (207.8, 77.3483) -> (206.5, 77)
  line L14 (206.5, 77) -> (204, 77)
  line L15 (204, 77) -> (204, 73.517)
  line L16 (204, 73.517) -> (203.233, 72.75)
  line L17 (203.233, 72.75) -> (200, 72.75)
  line L18 (200, 72.75) -> (200, 103.75)
  constraints: 38 end point, 4 point on circle, 2 centre point
revolve "Revolution26" add sketch "Sketch_14" angle 360 about axis through (200, 475, -72.75) along (0, 0, 1)
thread "Thread2" size "M8x1.25" class "6g" standard "ISO Metric profile" length 1.4216
sketch "Sketch_15" plane through (0, 25, 0) normal (0, 1, 0) x (1, 0, 0)
  line L0 (-200, 72.75) -> (-200, 103.75)
  line L1 (-200, 103.75) -> (-193.5, 103.75)
  line L2 (-193.5, 103.75) -> (-193.5, 102.75)
  line L3 (-193.5, 102.75) -> (-192.45, 102.75)
  line L4 (-192.45, 102.75) -> (-192.25, 102.55)
  line L5 (-192.25, 102.55) -> (-192.25, 93.55)
  arc A0 (-192.55, 93.25) -> (-192.25, 93.55) centre (-192.55, 93.55) ccw
  line L6 (-192.55, 93.25) -> (-192.25, 93.25)
  line L7 (-192.25, 93.25) -> (-192.25, 87.75)
  line L8 (-192.25, 87.75) -> (-196, 87.75)
  line L9 (-196, 87.75) -> (-196, 85)
  line L10 (-196, 85) -> (-191, 85)
  arc A1 (-190.8875, 82.5051) -> (-191, 85) centre (-191, 83.75) ccw
  line L11 (-190.8875, 82.5051) -> (-192.2, 82.3864)
  line L12 (-192.2, 82.3864) -> (-192.2, 77.3483)
  line L13 (-192.2, 77.3483) -> (-193.5, 77)
  line L14 (-193.5, 77) -> (-196, 77)
  line L15 (-196, 77) -> (-196, 73.517)
  line L16 (-196, 73.517) -> (-196.767, 72.75)
  line L17 (-196.767, 72.75) -> (-200, 72.75)
  line L18 (-200, 72.75) -> (-200, 103.75)
  constraints: 38 end point, 4 point on circle, 2 centre point
revolve "Revolution27" add sketch "Sketch_15" angle 360 about axis through (-200, 25, -72.75) along (0, 0, 1)
thread "Thread3" size "M8x1.25" class "6g" standard "ISO Metric profile" length 1.4216
sketch "Sketch_16" plane through (0, 25, 0) normal (0, 1, 0) x (1, 0, 0)
  line L0 (200, 72.75) -> (200, 103.75)
  line L1 (200, 103.75) -> (206.5, 103.75)
  line L2 (206.5, 103.75) -> (206.5, 102.75)
  line L3 (206.5, 102.75) -> (207.55, 102.75)
  line L4 (207.55, 102.75) -> (207.75, 102.55)
  line L5 (207.75, 102.55) -> (207.75, 93.55)
  arc A0 (207.45, 93.25) -> (207.75, 93.55) centre (207.45, 93.55) ccw
  line L6 (207.45, 93.25) -> (207.75, 93.25)
  line L7 (207.75, 93.25) -> (207.75, 87.75)
  line L8 (207.75, 87.75) -> (204, 87.75)
  line L9 (204, 87.75) -> (204, 85)
  line L10 (204, 85) -> (209, 85)
  arc A1 (209.1125, 82.5051) -> (209, 85) centre (209, 83.75) ccw
  line L11 (209.1125, 82.5051) -> (207.8, 82.3864)
  line L12 (207.8, 82.3864) -> (207.8, 77.3483)
  line L13 (207.8, 77.3483) -> (206.5, 77)
  line L14 (206.5, 77) -> (204, 77)
  line L15 (204, 77) -> (204, 73.517)
  line L16 (204, 73.517) -> (203.233, 72.75)
  line L17 (203.233, 72.75) -> (200, 72.75)
  line L18 (200, 72.75) -> (200, 103.75)
  constraints: 38 end point, 4 point on circle, 2 centre point
revolve "Revolution28" add sketch "Sketch_16" angle 360 about axis through (200, 25, -72.75) along (0, 0, 1)
thread "Thread4" size "M8x1.25" class "6g" standard "ISO Metric profile" length 1.4216
sketch "Sketch_100" plane through (0, 0, -76.75) normal (0, 0, 1) x (1, 0, 0)
  line L0 (-247.5, 497.5) -> (-247.5, 2.5)
  line L1 (-247.5, 2.5) -> (247.5, 2.5)
  line L2 (247.5, 2.5) -> (247.5, 497.5)
  line L3 (247.5, 497.5) -> (-247.5, 497.5)
  line L4 (193.5, 471.2472) -> (200, 467.4944)
  line L5 (200, 467.4944) -> (206.5, 471.2472)
  line L6 (206.5, 471.2472) -> (206.5, 478.7528)
  line L7 (206.5, 478.7528) -> (200, 482.5056)
  line L8 (200, 482.5056) -> (193.5, 478.7528)
  line L9 (193.5, 478.7528) -> (193.5, 471.2472)
  line L10 (193.5, 21.2472) -> (200, 17.4944)
  line L11 (200, 17.4944) -> (206.5, 21.2472)
  line L12 (206.5, 21.2472) -> (206.5, 28.7528)
  line L13 (206.5, 28.7528) -> (200, 32.5056)
  line L14 (200, 32.5056) -> (193.5, 28.7528)
  line L15 (193.5, 28.7528) -> (193.5, 21.2472)
  line L16 (-6.5, 471.2472) -> (0, 467.4944)
  line L17 (0, 467.4944) -> (6.5, 471.2472)
  line L18 (6.5, 471.2472) -> (6.5, 478.7528)
  line L19 (6.5, 478.7528) -> (0, 482.5056)
  line L20 (0, 482.5056) -> (-6.5, 478.7528)
  line L21 (-6.5, 478.7528) -> (-6.5, 471.2472)
  line L22 (-6.5, 21.2472) -> (0, 17.4944)
  line L23 (0, 17.4944) -> (6.5, 21.2472)
  line L24 (6.5, 21.2472) -> (6.5, 28.7528)
  line L25 (6.5, 28.7528) -> (0, 32.5056)
  line L26 (0, 32.5056) -> (-6.5, 28.7528)
  line L27 (-6.5, 28.7528) -> (-6.5, 21.2472)
  line L28 (-206.5, 471.2472) -> (-200, 467.4944)
  line L29 (-200, 467.4944) -> (-193.5, 471.2472)
  line L30 (-193.5, 471.2472) -> (-193.5, 478.7528)
  line L31 (-193.5, 478.7528) -> (-200, 482.5056)
  line L32 (-200, 482.5056) -> (-206.5, 478.7528)
  line L33 (-206.5, 478.7528) -> (-206.5, 471.2472)
  line L34 (-206.5, 21.2472) -> (-200, 17.4944)
  line L35 (-200, 17.4944) -> (-193.5, 21.2472)
  line L36 (-193.5, 21.2472) -> (-193.5, 28.7528)
  line L37 (-193.5, 28.7528) -> (-200, 32.5056)
  line L38 (-200, 32.5056) -> (-206.5, 28.7528)
  line L39 (-206.5, 28.7528) -> (-206.5, 21.2472)
  constraints: 80 end point
extrude "Extrusion23" cut sketch "Sketch_100" against normal blind 6
sketch "Sketch_139" plane through (0, 25, 0) normal (0, 1, 0) x (1, 0, 0)
  line L0 (-200, 81.6814) -> (-200, 85)
  line L1 (-200, 85) -> (-191, 85)
  arc A0 (-190.8875, 82.5051) -> (-191, 85) centre (-191, 83.75) ccw
  line L2 (-190.8875, 82.5051) -> (-200, 81.6814)
  line L3 (-200, 81.6814) -> (-200, 85)
  constraints: 8 end point, 2 point on circle, 1 centre point
revolve "Revolution29" add sketch "Sketch_139" angle 360 about axis through (-200, 25, -81.6814) along (0, 0, 1)
sketch "Sketch_140" plane through (0, 25, 0) normal (0, 1, 0) x (1, 0, 0)
  line L0 (200, 81.6814) -> (200, 85)
  line L1 (200, 85) -> (209, 85)
  arc A0 (209.1125, 82.5051) -> (209, 85) centre (209, 83.75) ccw
  line L2 (209.1125, 82.5051) -> (200, 81.6814)
  line L3 (200, 81.6814) -> (200, 85)
  constraints: 8 end point, 2 point on circle, 1 centre point
revolve "Revolution30" add sketch "Sketch_140" angle 360 about axis through (200, 25, -81.6814) along (0, 0, 1)
sketch "Sketch54" plane through (229.5, 20.5, 96.3319) normal (1, 0, 0) x (0, 0, -1)
  point P0 (7.0819, 417)
hole "Hole1" at (229.5, 437.5, 89.25) direction (-1, 0, 0) diameter 6.5 depth 1.25
sketch "Sketch55" plane through (229.5, 20.5, 96.3319) normal (1, 0, 0) x (0, 0, -1)
  point P0 (7.0819, 42)
hole "Hole2" at (229.5, 62.5, 89.25) direction (-1, 0, 0) diameter 6.5 depth 1.25
sketch "Sketch56" plane through (-229.5, 20.5, 83.25) normal (-1, 0, 0) x (0, 0, 1)
  point P0 (6, 417)
hole "Hole3" at (-229.5, 437.5, 89.25) direction (1, 0, 0) diameter 6.5 depth 1.25
sketch "Sketch57" plane through (-229.5, 20.5, 83.25) normal (-1, 0, 0) x (0, 0, 1)
  point P0 (6, 42)
hole "Hole4" at (-229.5, 62.5, 89.25) direction (1, 0, 0) diameter 6.5 depth 1.25
sketch "Sketch_27" plane through (0, 0, 0) normal (0, 1, 0) x (1, 0, 0)
  line L0 (-246.25, -78.25) -> (246.25, -78.25)
  line L1 (246.25, -78.25) -> (246.25, 101.25)
  line L2 (246.25, 101.25) -> (-246.25, 101.25)
  line L3 (-246.25, 101.25) -> (-246.25, -78.25)
  constraints: 8 end point
extrude "Extrusion24" cut sketch "Sketch_27" along normal blind 1.25
sketch "Sketch_28" plane through (0, 0, 0) normal (0, 1, 0) x (1, 0, 0)
  line L0 (-246.25, -78.25) -> (246.25, -78.25)
  line L1 (246.25, -78.25) -> (246.25, 101.25)
  line L2 (246.25, 101.25) -> (-246.25, 101.25)
  line L3 (-246.25, 101.25) -> (-246.25, -78.25)
  arc A0 (-230.5, -31) -> (-191.5, -70) centre (-191.5, -31) ccw
  line L4 (-191.5, -70) -> (191.5, -70)
  arc A1 (191.5, -70) -> (230.5, -31) centre (191.5, -31) ccw
  line L5 (230.5, -31) -> (230.5, 54)
  arc A2 (230.5, 54) -> (191.5, 93) centre (191.5, 54) ccw
  line L6 (191.5, 93) -> (-191.5, 93)
  arc A3 (-191.5, 93) -> (-230.5, 54) centre (-191.5, 54) ccw
  line L7 (-230.5, 54) -> (-230.5, -31)
  circle A4 centre (-233.5, -65.5) radius 8
  constraints: 16 end point, 8 point on circle, 5 centre point
extrude "Extrusion25" add sketch "Sketch_28" along normal blind 1.25
sketch "Sketch_29" plane through (0, 0, 0) normal (1, 0, 0) x (0, 0, -1)
  line L0 (68, 4) -> (84.6651, 4)
  line L1 (84.6651, 4) -> (91.5933, 0)
  line L2 (91.5933, 0) -> (93, 0)
  line L3 (93, 0) -> (93, 1.25)
  line L4 (93, 1.25) -> (91.9282, 1.25)
  line L5 (91.9282, 1.25) -> (85, 5.25)
  line L6 (85, 5.25) -> (68, 5.25)
  line L7 (68, 5.25) -> (68, 4)
  constraints: 16 end point
extrude "Extrusion26" add sketch "Sketch_29" along normal mid plane 383
sketch "Sketch_30" plane through (0, 0, 0) normal (1, 0, 0) x (0, 0, -1)
  line L0 (-70, 0) -> (-68.5933, 0)
  line L1 (-68.5933, 0) -> (-61.6651, 4)
  line L2 (-61.6651, 4) -> (-45, 4)
  line L3 (-45, 4) -> (-45, 5.25)
  line L4 (-45, 5.25) -> (-62, 5.25)
  line L5 (-62, 5.25) -> (-68.9282, 1.25)
  line L6 (-68.9282, 1.25) -> (-70, 1.25)
  line L7 (-70, 1.25) -> (-70, 0)
  constraints: 16 end point
extrude "Extrusion27" add sketch "Sketch_30" along normal mid plane 383
sketch "Sketch_31" plane through (191.5, 0, 0) normal (1, 0, 0) x (0, 0, -1)
  line L0 (54, 4) -> (54, 5.25)
  line L1 (68, 4) -> (84.6651, 4)
  line L2 (84.6651, 4) -> (91.5933, 0)
  line L3 (91.5933, 0) -> (95, 0)
  line L4 (95, 0) -> (95, 1.25)
  line L5 (95, 1.25) -> (91.9282, 1.25)
  line L6 (91.9282, 1.25) -> (85, 5.25)
  line L7 (85, 5.25) -> (68, 5.25)
  line L8 (68, 5.25) -> (68, 4)
  constraints: 18 end point
revolve "Revolution31" add sketch "Sketch_31" angle 90 about axis through (191.5, 4, -54) along (0, -1, 0)
sketch "Sketch_32" plane through (191.5, 0, 0) normal (1, 0, 0) x (0, 0, -1)
  line L0 (-31, 5.25) -> (-31, 4)
  line L1 (-72, 0) -> (-68.5933, 0)
  line L2 (-68.5933, 0) -> (-61.6651, 4)
  line L3 (-61.6651, 4) -> (-45, 4)
  line L4 (-45, 4) -> (-45, 5.25)
  line L5 (-45, 5.25) -> (-62, 5.25)
  line L6 (-62, 5.25) -> (-68.9282, 1.25)
  line L7 (-68.9282, 1.25) -> (-72, 1.25)
  line L8 (-72, 1.25) -> (-72, 0)
  constraints: 18 end point
revolve "Revolution32" add sketch "Sketch_32" angle 90 about axis through (191.5, 5.25, 31) along (0, 1, 0)
sketch "Sketch_33" plane through (-191.5, 0, 0) normal (1, 0, 0) x (0, 0, -1)
  line L0 (54, 4) -> (54, 5.25)
  line L1 (68, 4) -> (84.6651, 4)
  line L2 (84.6651, 4) -> (91.5933, 0)
  line L3 (91.5933, 0) -> (95, 0)
  line L4 (95, 0) -> (95, 1.25)
  line L5 (95, 1.25) -> (91.9282, 1.25)
  line L6 (91.9282, 1.25) -> (85, 5.25)
  line L7 (85, 5.25) -> (68, 5.25)
  line L8 (68, 5.25) -> (68, 4)
  constraints: 18 end point
revolve "Revolution33" add sketch "Sketch_33" angle 90 about axis through (-191.5, 4, -54) along (0, 1, 0)
sketch "Sketch_34" plane through (-191.5, 0, 0) normal (1, 0, 0) x (0, 0, -1)
  line L0 (-31, 5.25) -> (-31, 4)
  line L1 (-72, 0) -> (-68.5933, 0)
  line L2 (-68.5933, 0) -> (-61.6651, 4)
  line L3 (-61.6651, 4) -> (-45, 4)
  line L4 (-45, 4) -> (-45, 5.25)
  line L5 (-45, 5.25) -> (-62, 5.25)
  line L6 (-62, 5.25) -> (-68.9282, 1.25)
  line L7 (-68.9282, 1.25) -> (-72, 1.25)
  line L8 (-72, 1.25) -> (-72, 0)
  constraints: 18 end point
revolve "Revolution34" add sketch "Sketch_34" angle 90 about axis through (-191.5, 5.25, 31) along (0, -1, 0)
sketch "Sketch_35" plane through (0, 0, -11.5) normal (0, 0, 1) x (1, 0, 0)
  line L0 (205.5, 4) -> (222.1651, 4)
  line L1 (222.1651, 4) -> (229.0933, 0)
  line L2 (229.0933, 0) -> (230.5, 0)
  line L3 (230.5, 0) -> (230.5, 1.25)
  line L4 (230.5, 1.25) -> (229.4282, 1.25)
  line L5 (229.4282, 1.25) -> (222.5, 5.25)
  line L6 (222.5, 5.25) -> (205.5, 5.25)
  line L7 (205.5, 5.25) -> (205.5, 4)
  constraints: 16 end point
extrude "Extrusion28" add sketch "Sketch_35" along normal mid plane 85
sketch "Sketch_36" plane through (0, 0, -11.5) normal (0, 0, 1) x (1, 0, 0)
  line L0 (-230.5, 0) -> (-229.0933, 0)
  line L1 (-229.0933, 0) -> (-222.1651, 4)
  line L2 (-222.1651, 4) -> (-205.5, 4)
  line L3 (-205.5, 4) -> (-205.5, 5.25)
  line L4 (-205.5, 5.25) -> (-222.5, 5.25)
  line L5 (-222.5, 5.25) -> (-229.4282, 1.25)
  line L6 (-229.4282, 1.25) -> (-230.5, 1.25)
  line L7 (-230.5, 1.25) -> (-230.5, 0)
  constraints: 16 end point
extrude "Extrusion29" add sketch "Sketch_36" along normal mid plane 85
sketch "Sketch_37" plane through (0, 5.25, 0) normal (0, 1, 0) x (1, 0, 0)
  arc A0 (-220.5, -32) -> (-192.5, -60) centre (-192.5, -32) ccw
  line L0 (-192.5, -60) -> (192.5, -60)
  arc A1 (192.5, -60) -> (220.5, -32) centre (192.5, -32) ccw
  line L1 (220.5, -32) -> (220.5, 55)
  arc A2 (220.5, 55) -> (192.5, 83) centre (192.5, 55) ccw
  line L2 (192.5, 83) -> (-192.5, 83)
  arc A3 (-192.5, 83) -> (-220.5, 55) centre (-192.5, 55) ccw
  line L3 (-220.5, 55) -> (-220.5, -32)
  constraints: 8 end point, 8 point on circle, 4 centre point
extrude "Extrusion30" cut sketch "Sketch_37" against normal blind 1.25